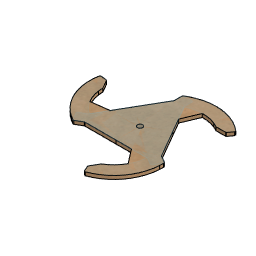
Hook Wheel Full Size v5 (Autodesk Fusion 360 design; units mm, degrees)
Autodesk Fusion 360 part; units mm, degrees
sketch "Sketch1" plane through (0, 0, 0) normal (0, 0, 1) x (1, 0, 0)
  line L0 (0, 0) -> (140, 0) construction
  line L1 (-106.226913, -44.00959) -> (-15, 114)
  line L2 (15, 114) -> (106.226913, -44.00959)
  line L3 (91.226896, -69.990381) -> (-91.226896, -69.990381)
  line L4 (-15, 140) -> (15, 140)
  line L5 (15, 140) -> (15, 114)
  line L6 (-15, 114) -> (-15, 140)
  line L7 (15, 140) -> (14.270763, 139.270763) construction
  line L8 (-128.743557, -57.009619) -> (-106.226913, -44.00959)
  line L9 (-113.743557, -82.990381) -> (-128.743557, -57.009619)
  line L10 (-91.226896, -69.990381) -> (-113.743557, -82.990381)
  line L11 (113.743557, -82.990381) -> (91.226896, -69.990381)
  line L12 (128.743557, -57.009619) -> (113.743557, -82.990381)
  line L13 (106.226913, -44.00959) -> (128.743557, -57.009619)
  dimension "d5" = 30
  dimension "d6" = 26
  dimension "d7" = 26
  dimension "d8" = 26
  dimension "d9" = 30
  dimension "d10" = 26
  dimension "d11" = 30
  dimension "d12" = 26
  dimension "d13" = 26
  constraint horizontal L0
  constraint coincident L0.start origin
  constraint horizontal L3
  constraint horizontal L4
  constraint perpendicular L4 L5
  constraint parallel L5 L6
  measures "d5" distance of L4.start L4.end
  measures "d6" distance of L4.end L2.start
  measures "d7" distance of L4.start L1.end
extrude "Extrude1" add sketch "Sketch1" along normal blind 10 makes body 1
fillet "Fillet1" radius 3 12 edges at (-113.743557, -82.990381, 5) (-91.226896, -69.990381, 5) (91.226896, -69.990381, 5) (113.743557, -82.990381, 5) (-128.743557, -57.009619, 5) (-106.226913, -44.00959, 5) (-15, 114, 5) (-15, 140, 5) (15, 140, 5) (15, 114, 5) (106.226913, -44.00959, 5) (128.743557, -57.009619, 5) on bodies 1
sketch "Sketch2" plane through (0, 0, 0) normal (0, 0, 1) x (1, 0, 0)
  line L0 (240.661595, 203.529107) -> (270, 203.529107)
  line L1 (270, 203.529107) -> (282.347572, 220.223219)
  line L2 (139.338405, 203.529107) -> (115.946551, 203.529107)
  line L3 (115.946551, 203.529107) -> (115.946551, 233.811139)
  arc A0 (240.661595, 203.529107) -> (139.338405, 203.529107) centre (190, 115) ccw
  arc A1 (282.347572, 220.223219) -> (115.946551, 233.811139) centre (190, 115) ccw
  dimension "d18" = 280
  constraint horizontal L0
  constraint parallel L0 L2
  constraint perpendicular L2 L3
  constraint concentric A0 A1
  measures "d18" diameter of A1
extrude "Extrude2" add sketch "Sketch2" along normal blind 10 separate body makes body 2
fillet "Fillet2" radius 3 2 edges at (115.946551, 203.529107, 5) (282.347572, 220.223219, 5) on bodies 2
sketch "Sketch3" plane through (0, 0, 10) normal (0, 0, 1) x (-1, 0, 0)
  arc A0 (-127.243558, 59.607692) -> (-126.145486, 55.509618) centre (-124.645482, 58.107692) ccw
  line L0 (-126.145486, 55.509618) -> (-106.923063, 44.411514)
  arc A1 (-105.82499, 43.31344) -> (-106.923063, 44.411514) centre (-108.423066, 41.813439) ccw
  line L1 (-105.82499, 43.31344) -> (-15.401924, -113.303847)
  arc A2 (-15, -114.803848) -> (-15.401924, -113.303847) centre (-18, -114.803848) ccw
  line L2 (-15, -114.803848) -> (-15, -137)
  arc A3 (-15, -137) -> (-12, -140) centre (-12, -137) ccw
  line L3 (-12, -140) -> (12, -140)
  arc A4 (12, -140) -> (15, -137) centre (12, -137) ccw
  line L4 (15, -137) -> (15, -114.803848)
  arc A5 (15.401924, -113.303847) -> (15, -114.803848) centre (18, -114.803848) ccw
  line L5 (15.401924, -113.303847) -> (105.82499, 43.31344)
  arc A6 (106.923063, 44.411514) -> (105.82499, 43.31344) centre (108.423066, 41.813439) ccw
  line L6 (106.923063, 44.411514) -> (126.145486, 55.509618)
  arc A7 (126.145486, 55.509618) -> (127.243558, 59.607692) centre (124.645482, 58.107692) ccw
  line L7 (127.243558, 59.607692) -> (115.243557, 80.392305)
  arc A8 (115.243557, 80.392305) -> (111.14548, 81.490381) centre (112.64548, 78.892305) ccw
  line L8 (111.14548, 81.490381) -> (91.923048, 70.392305)
  arc A9 (90.423048, 69.990381) -> (91.923048, 70.392305) centre (90.423048, 72.990381) ccw
  line L9 (90.423048, 69.990381) -> (-90.423048, 69.990381)
  arc A10 (-91.923048, 70.392305) -> (-90.423048, 69.990381) centre (-90.423048, 72.990381) ccw
  line L10 (-91.923048, 70.392305) -> (-111.14548, 81.490381)
  arc A11 (-111.14548, 81.490381) -> (-115.243557, 80.392305) centre (-112.64548, 78.892305) ccw
  line L11 (-115.243557, 80.392305) -> (-127.243558, 59.607692)
move_body "Move1" bodies 2 to x (1, 0, 0) y (0, 1, 0) z (0, 0, 1) at (0, -85, 0)
fillet "Fillet3" radius 1 2 edges at (240.661595, 118.529107, 5) (270, 118.529107, 5) on bodies 2
pattern_circular "C-Pattern1" count 3 over 360 about axis through (0, 0, 1.75) along (0, 0, 1) of bodies 2 makes body 3 at (-240.465128, 159.404932, 0) makes body 4 at (-17.816156, -287.951375, 0)
move_body "Move2" bodies 2 to x (1, 0, 0) y (0, 1, 0) z (0, 0, 1) at (-130, -10, 0)
move_body "Move3" bodies 4 to x (1, 0, 0) y (0, 1, 0) z (0, 0, 1) at (56.5, 116.5, 0)
move_body "Move4" bodies 2 to x (1, 0, 0) y (0, 1, 0) z (0, 0, 1) at (0.9, 0.8, 0)
move_body "Move5" bodies 3 to x (1, 0, 0) y (0, 1, 0) z (0, 0, 1) at (72.6, -107.2, 0)
move_body "Move6" bodies 2 to x (1, 0, 0) y (0, 1, 0) z (0, 0, 1) at (-0.09, -0.1, 0)
combine "Combine1" operation add target body 3 tool bodies 1
combine "Combine2" operation add target body 4 tool bodies 3
combine "Combine3" operation add target body 2 tool bodies 4
sketch "Sketch5" plane through (0, 0, 10) normal (0, 0, 1) x (-1, 0, 0)
  circle A0 centre (0, 0) radius 7.5
  dimension "d40" = 15
  constraint coincident A0.centre origin
  measures "d40" diameter of A0
extrude "Extrude7" cut sketch "Sketch5" against normal blind 10 bodies 2
sketch "Sketch1 (2)" plane through (0, 0, 10) normal (0, 0, 1) x (-1, 0, 0) in component "Component"
  circle A0 centre (0, 0) radius 7.5
  arc A1 (-111.242365, -109.359893) -> (-15.972048, -112.316364) centre (-60.81, -20.7) ccw
  arc A2 (-111.242365, -109.359893) -> (-111.7368, -109.229107) centre (-111.7368, -110.229107) ccw
  line L0 (-111.7368, -109.229107) -> (-140.305827, -109.229107)
  arc A3 (-140.305827, -109.229107) -> (-141.109809, -109.634453) centre (-140.305827, -110.229107) ccw
  line L1 (-141.109809, -109.634453) -> (-151.500099, -123.68229)
  arc A4 (-151.500099, -123.68229) -> (-151.021252, -127.760403) centre (-149.088154, -125.466252) ccw
  arc A5 (-151.021252, -127.760403) -> (12.530108, -139.952793) centre (-60.81, -20.7) ccw
  arc A6 (12.530108, -139.952793) -> (15, -137) centre (12, -137) ccw
  line L2 (15, -137) -> (15, -114.803848)
  arc A7 (15.401924, -113.303847) -> (15, -114.803848) centre (18, -114.803848) ccw
  line L3 (15.401924, -113.303847) -> (105.255344, 42.326785)
  arc A8 (150.378664, -41.69059) -> (105.255344, 42.326785) centre (48.380762, -42.344827) ccw
  arc A9 (150.378664, -41.69059) -> (150.512618, -42.184176) centre (151.378643, -41.684176) ccw
  line L4 (150.512618, -42.184176) -> (164.797131, -66.925679)
  arc A10 (164.797131, -66.925679) -> (165.550162, -67.419274) centre (165.663157, -66.425679) ccw
  line L5 (165.550162, -67.419274) -> (182.911091, -69.393612)
  arc A11 (182.911091, -69.393612) -> (186.203417, -66.939861) centre (183.250075, -66.412825) ccw
  arc A12 (186.203417, -66.939861) -> (114.945804, 80.818054) centre (48.380762, -42.344827) ccw
  arc A13 (114.945804, 80.818054) -> (111.14548, 81.490381) centre (112.64548, 78.892305) ccw
  line L6 (111.14548, 81.490381) -> (91.923048, 70.392305)
  arc A14 (90.423048, 69.990381) -> (91.923048, 70.392305) centre (90.423048, 72.990381) ccw
  line L7 (90.423048, 69.990381) -> (-89.244013, 69.990381)
  arc A15 (-39.046299, 151.050482) -> (-89.244013, 69.990381) centre (12.519238, 63.044827) ccw
  arc A16 (-39.046299, 151.050482) -> (-38.685818, 151.413283) centre (-39.551843, 151.913283) ccw
  line L8 (-38.685818, 151.413283) -> (-24.401304, 176.154786)
  arc A17 (-24.401304, 176.154786) -> (-24.350354, 177.053727) centre (-25.26733, 176.654786) ccw
  line L9 (-24.350354, 177.053727) -> (-31.320991, 193.075901)
  arc A18 (-31.320991, 193.075901) -> (-35.092165, 194.700265) centre (-34.071921, 191.879077) ccw
  arc A19 (-35.092165, 194.700265) -> (-127.428706, 59.227364) centre (12.519238, 63.044827) ccw
  arc A20 (-127.428706, 59.227364) -> (-126.145486, 55.509618) centre (-124.645482, 58.107692) ccw
  line L10 (-126.145486, 55.509618) -> (-106.923063, 44.411514)
  arc A21 (-105.82499, 43.31344) -> (-106.923063, 44.411514) centre (-108.423066, 41.813439) ccw
  line L11 (-105.82499, 43.31344) -> (-15.972048, -112.316364)
extrude "Extrude2'" add sketch "Sketch1 (2)" against normal blind 6 separate body makes body 5 in component "Component"
combine "Combine4" operation add target body 2 tool bodies 5
sketch "Sketch6" plane through (0, 0, 10) normal (0, 0, 1) x (-1, 0, 0)
  line L0 (-45, 70) -> (-77.000001, 112.000002)
  line L1 (-45, 70) -> (-72.867767, 59.925039)
  line L2 (-72.867767, 59.925039) -> (-97.850641, 64.962519)
  line L3 (-97.850641, 64.962519) -> (-91.651047, 95.708776)
  line L4 (-91.651047, 95.708776) -> (-77.000001, 112.000002)
  constraint perpendicular L2 L3
extrude "Extrude8" add sketch "Sketch6" against normal blind 10 bodies 2
pattern_circular "C-Pattern2" count 3 over 360 about axis through (0, 0, 1.75) along (0, 0, 1) of bodies 2 makes body 6 at (114.447446, -122.1399, 6.666667) makes body 7 at (124.061467, 145.649881, 6.666667)
combine "Combine5" operation add target body 7 tool bodies 2
combine "Combine6" operation add target body 6 tool bodies 7
component "Component" placed x (1, 0, 0) y (0, 1, 0) z (0, 0, 1) at (0, 0, 0)
